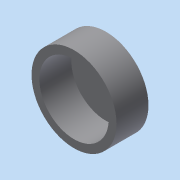
# Autodesk Inventor part: wheel
Saved by Autodesk Inventor 2015 (Build 190159000, 159)
## iProperties
Created: 2015-06-23
Part Number: wheel
Material: Generic
Document SubType Name: Modeling
Designer: Rahul
Density: 1 g/cm^3
Appearance: Default
Author: Rahul
Autodesk Inventor part; units mm, degrees
ref_plane "YZ Plane" through (0, 0, 0) normal (1, 0, 0) x (0, 1, 0)
ref_plane "XZ Plane" through (0, 0, 0) normal (0, 1, 0) x (-1, 0, 0)
ref_plane "XY Plane" through (0, 0, 0) normal (0, 0, 1) x (1, 0, 0)
sketch "Sketch1" plane through (0, 0, 0) normal (0, 0, 1) x (1, 0, 0)
  circle A0 centre (0, 0) radius 42.5
  dimension "d0" = 85
  constraints: 1 centre point, 1 coincident
  measures "d0" diameter of A0
extrude "Extrusion1" add sketch "Sketch1" along normal blind 31.93
sketch "Sketch2" plane through (0, 0, 31.93) normal (0, 0, 1) x (1, 0, 0)
  circle A0 centre (0, 0) radius 34.67
  circle A1 centre (0, 0) radius 42.5 projected
  dimension "d3" = 7.83
  constraints: 1 centre point, 1 coincident
  measures "d3" radial gap between concentric circles of A1 A0
extrude "Extrusion2" cut sketch "Sketch2" against normal blind 31.92 contours A0
sketch "Sketch5" plane through (0, 0, 0.01) normal (0, 0, 1) x (1, 0, 0)
  line L0 (3.2417, 5.6147) -> (6.4833, 0)
  line L1 (6.4833, 0) -> (3.2417, -5.6147)
  line L2 (3.2417, -5.6147) -> (-3.2417, -5.6147)
  line L3 (-3.2417, -5.6147) -> (-6.4833, 0)
  line L4 (-6.4833, 0) -> (-3.2417, 5.6147)
  line L5 (-3.2417, 5.6147) -> (3.2417, 5.6147)
  line L6 (-59.5, 0) -> (59.5, 0) projected
  line L7 (0, -59.5) -> (0, 59.5) projected
  circle A0 centre (0, 0) radius 6.4833
  circle A1 centre (0, 0) radius 8.1344
  dimension "d13" = 12.9667
  dimension "d14" = 1.651
  constraints: 12 end point, 3 coincident, 1 centre point, 17 other
  measures "d13" distance of L0.end L3.end
extrude "Extrusion5" add sketch "Sketch5" along normal blind 3.0734 contours A0 L0 | A0 L7 A1 L6 | L5 L7 A0 | A0 L1 | L6 A1 L7 A0 | L5 A0 L7 | A0 L6 A1 L7 | A0 L7 L2 | L4 A0 | L7 A0 L2 | L7 A1 L6 A0 | L3 A0
body "Solid1"
